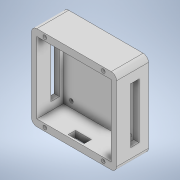
# Autodesk Inventor part: Case_Base
Saved by Autodesk Inventor 2022 (Build 260153000, 153)
## iProperties
Created: 2024-06-23
Part Number: Case_Base
Material: Типовые
Document SubType Name: Modeling
Designer: Timur
Density: 1 g/cm^3
Appearance: По умолчанию
Author: Timur
Autodesk Inventor part; units mm, degrees
ref_plane "YZ Plane" through (0, 0, 0) normal (1, 0, 0) x (0, 1, 0)
ref_plane "XZ Plane" through (0, 0, 0) normal (0, 1, 0) x (-1, 0, 0)
ref_plane "XY Plane" through (0, 0, 0) normal (0, 0, 1) x (1, 0, 0)
sketch "Эскиз1" plane through (0, 0, 0) normal (0, 0, 1) x (1, 0, 0)
  circle A0 centre (0, 2.5) radius 1.1
  circle A1 centre (55, 2.5) radius 1.1
  circle A2 centre (0, 57.5) radius 1.1
  circle A3 centre (55, 57.5) radius 1.1
  line L0 (15.5, 60) -> (0, 60)
  line L1 (-2.5, 57.5) -> (-2.5, 2.5)
  line L2 (55, 60) -> (39.5, 60)
  line L3 (57.5, 2.5) -> (57.5, 57.5)
  line L4 (-2.5, 2.5) -> (-2.5, 0)
  line L5 (0, 60) -> (-2.5, 60)
  line L6 (-2.5, 60) -> (-2.5, 57.5)
  line L7 (39.5, 60) -> (15.5, 60)
  line L8 (57.5, 2.5) -> (57.5, 0)
  line L9 (57.5, 0) -> (-2.5, 0)
  line L10 (57.5, 57.5) -> (57.5, 60)
  line L11 (57.5, 60) -> (55, 60)
  line L12 (-7.5, 63.5411) -> (62.5, 63.5411)
  line L13 (62.5, 63.5411) -> (62.5, -3.5411)
  line L14 (62.5, -3.5411) -> (-7.5, -3.5411)
  line L15 (-7.5, -3.5411) -> (-7.5, 63.5411)
  line L16 (-7.5, 63.5411) -> (62.5, -3.5411) construction
  line L17 (62.5, 63.5411) -> (-7.5, -3.5411) construction
  point P0 (0, 0)
  point P1 (27.5, 30)
  dimension "d0" = 70
  constraints: 36 end point, 5 perpendicular, 4 centre point, 3 vertical, 2 horizontal, 2 midpoint, 2 parallel
  measures "d0" distance of L13.end L14.end
extrude "Выдавливание1" add sketch "Эскиз1" along normal blind 5 contours A0 | A1 | A2 | A3 | L7 L2 L11 L10 L3 L8 L9 L4 L1 L6 L5 L0 | L12 L13 L14 L15
sketch "Эскиз2" plane through (0, 0, 0) normal (0, 0, -1) x (-1, 0, 0)
  line L0 (7.5, 63.5411) -> (7.5, -3.5411) projected
  line L1 (-62.5, -3.5411) -> (-62.5, 63.5411) projected
  line L2 (-62.5, 63.5411) -> (7.5, 63.5411) projected
  line L3 (7.5, -3.5411) -> (-62.5, -3.5411) projected
  line L4 (12.5, 70) -> (-67.5, 70)
  line L5 (-67.5, 70) -> (-67.5, -10)
  line L6 (-67.5, -10) -> (12.5, -10)
  line L7 (12.5, -10) -> (12.5, 70)
  line L8 (12.5, 70) -> (-67.5, -10) construction
  line L9 (-67.5, 70) -> (12.5, -10) construction
  point P0 (0, 0)
  point P1 (-27.5, 30)
  dimension "d3" = 80
  dimension "d4" = 80
  constraints: 12 end point, 2 midpoint, 2 parallel, 1 horizontal, 1 perpendicular
  measures "d3" distance of L6.end L5.end
  measures "d4" distance of L5.end L4.end
extrude "Выдавливание2" add sketch "Эскиз2" against normal blind 30
sketch "Эскиз3" plane through (0, 0, 5) normal (0, 0, 1) x (1, 0, 0)
  circle A0 centre (55, 2.5) radius 1.75
  circle A1 centre (55, 57.5) radius 1.75
  circle A2 centre (0, 57.5) radius 1.75
  circle A3 centre (0, 2.5) radius 1.75
  point P0 (0, 0)
  dimension "d7" = 3.5
  dimension "d8" = 3.5
  dimension "d9" = 3.5
  dimension "d10" = 3.5
  constraints: 4 centre point, 4 coincident
  measures "d7" diameter of A0
  measures "d8" diameter of A1
  measures "d9" diameter of A2
  measures "d10" diameter of A3
extrude "Выдавливание3" cut sketch "Эскиз3" against normal blind 4
fillet "Сопряжение1" radius 5 4 edges at (67.5, -10, 15) (67.5, 70, 15) (-12.5, -10, 15) (-12.5, 70, 15)
sketch "Эскиз5" plane through (0, 0, 30) normal (0, 0, 1) x (1, 0, 0)
  circle A0 centre (0, 57.5) radius 1.75 projected
  line L0 (0, 57.5) -> (0, 63.5411)
  line L1 (62.5, 63.5411) -> (-7.5, 63.5411) projected
  line L2 (-7.5, 70) -> (62.5, 70) projected
  line L3 (0, 70) -> (0, 63.5411)
  circle A1 centre (55, 57.5) radius 1.75 projected
  line L4 (55, 57.5) -> (55, 63.5411)
  line L5 (55, 63.5411) -> (55, 70)
  circle A2 centre (55, 66.7706) radius 1.75
  circle A3 centre (0, 66.7706) radius 1.75
  circle A4 centre (55, 2.5) radius 1.75 projected
  line L6 (55, 2.5) -> (55, -3.5411)
  line L7 (62.5, -3.5411) -> (-7.5, -3.5411) projected
  line L8 (55, -3.5411) -> (55, -10)
  line L9 (62.5, -10) -> (-7.5, -10) projected
  circle A5 centre (0, 2.5) radius 1.75 projected
  line L10 (0, 2.5) -> (0, -3.5411)
  line L11 (0, -3.5411) -> (0, -10)
  circle A6 centre (55, -6.7706) radius 1.75
  circle A7 centre (0, -6.7706) radius 1.75
  point P0 (0, 0)
  dimension "d14" = 3.5
  dimension "d15" = 3.5
  dimension "d16" = 3.5
  dimension "d17" = 3.5
  constraints: 16 end point, 8 point on line, 4 centre point, 4 midpoint, 4 vertical, 1 perpendicular
  measures "d14" diameter of A2
  measures "d15" diameter of A3
  measures "d16" diameter of A6
  measures "d17" diameter of A7
extrude "Выдавливание4" cut sketch "Эскиз5" against normal blind 4 contours A3 L3 | L3 A3 | A2 L5 | L5 A2 | A6 L8 | L8 A6 | A7 L11 | L11 A7
sketch "Эскиз6" plane through (0, 0, 30) normal (0, 0, 1) x (1, 0, 0)
  line L0 (62.5, 70) -> (-7.5, 70) projected
  line L1 (-12.5, 65) -> (-12.5, -5) projected
  arc A0 (-7.5, 70) -> (-12.5, 65) centre (-7.5, 65) ccw projected
  arc A1 (67.5, 65) -> (62.5, 70) centre (62.5, 65) ccw projected
  line L2 (67.5, -5) -> (67.5, 65) projected
  arc A2 (62.5, -10) -> (67.5, -5) centre (62.5, -5) ccw projected
  line L3 (-7.5, -10) -> (62.5, -10) projected
  arc A3 (-12.5, -5) -> (-7.5, -10) centre (-7.5, -5) ccw projected
  circle A4 centre (0, 66.7706) radius 1.75 projected
  circle A5 centre (55, 66.7706) radius 1.75 projected
  circle A6 centre (55, -6.7706) radius 1.75 projected
  circle A7 centre (0, -6.7706) radius 1.75 projected
  line L4 (62.5, -3.5411) -> (-7.5, -3.5411) projected
  line L5 (-7.5, -3.5411) -> (-7.5, 63.5411) projected
  line L6 (-7.5, 63.5411) -> (62.5, 63.5411) projected
  line L7 (62.5, 63.5411) -> (62.5, -3.5411) projected
  point P0 (0, 0)
sketch "Эскиз7" plane through (67.5, -5, 0) normal (1, 0, 0) x (0, 0, -1)
  line L0 (-30, -5) -> (0, -5)
  line L1 (-30, 0) -> (-30, 70)
  line L2 (0, 75) -> (-30, 75)
  line L3 (0, 70) -> (0, 0)
  line L4 (-30, 35) -> (0, 35)
  line L5 (-12.99, 13.983) -> (-12.99, 13.543)
  line L6 (-12.55, 13.543) -> (-12.55, 13.983)
  line L7 (-12.99, 13.763) -> (-12.55, 13.763)
  line L8 (-13.44, 12.493) -> (-12.1, 12.493)
  line L9 (-16.77, 9) -> (-8.77, 9)
  line L10 (-8.77, 9) -> (-8.77, 61)
  line L11 (-8.77, 61) -> (-16.77, 61)
  line L12 (-16.77, 61) -> (-16.77, 9)
  line L13 (-12.77, 13.763) -> (-12.77, 10.2135)
  point P0 (0, 5)
  dimension "d20" = 26
  dimension "d21" = 26
  dimension "d22" = 8
  dimension "d23" = 4
  constraints: 28 end point, 5 midpoint, 2 parallel, 1 horizontal, 1 perpendicular, 1 vertical
  measures "d20" distance between parallel lines of L4 L9
  measures "d21" distance between parallel lines of L4 L11
  measures "d22" distance between parallel lines of L10 L12
  measures "d23" distance between parallel lines of L13 L12
extrude "Выдавливание5" cut sketch "Эскиз7" against normal through all
sketch "Эскиз8" plane through (-7.5, -10, 0) normal (0, -1, 0) x (1, 0, 0)
  line L0 (32, 26.125) -> (38, 26.125)
  line L1 (34.72, 23.225) -> (32.7, 23.225)
  line L2 (30.9, 24.9) -> (30.9, 25.1)
  line L3 (39.1, 25.1) -> (39.1, 24.9)
  line L4 (30.9, 25.1) -> (30.9, 26.125)
  line L5 (30.9, 26.125) -> (39.1, 26.125)
  line L6 (39.1, 26.125) -> (39.1, 23.225)
  line L7 (39.1, 23.225) -> (30.9, 23.225)
  line L8 (30.9, 23.225) -> (30.9, 25.1)
  line L9 (42.5, 20.675) -> (27.5, 20.675)
  line L10 (27.5, 20.675) -> (27.5, 28.675)
  line L11 (27.5, 28.675) -> (42.5, 28.675)
  line L12 (42.5, 28.675) -> (42.5, 20.675)
  line L13 (42.5, 20.675) -> (27.5, 28.675) construction
  line L14 (27.5, 20.675) -> (42.5, 28.675) construction
  line L15 (42.5, 21.175) -> (27.5, 21.175)
  line L16 (27.5, 21.175) -> (27.5, 28.175)
  line L17 (27.5, 28.175) -> (42.5, 28.175)
  line L18 (42.5, 28.175) -> (42.5, 21.175)
  line L19 (42.5, 21.175) -> (27.5, 28.175) construction
  line L20 (27.5, 21.175) -> (42.5, 28.175) construction
  point P0 (7.5, 0)
  point P1 (35, 24.675)
  dimension "d26" = 15
  dimension "d27" = 8
  dimension "d28" = 15
  dimension "d29" = 7
  constraints: 42 end point, 5 perpendicular, 4 midpoint, 4 parallel, 2 horizontal, 2 point on line, 1 vertical
  measures "d26" distance of L10.end L11.end
  measures "d27" distance of L9.end L10.end
  measures "d28" distance of L16.end L17.end
  measures "d29" distance of L15.end L16.end
extrude "Выдавливание6" cut sketch "Эскиз8" against normal blind 10 contours L0 L5 L6 L3 L7 L1 L8 L2 L4 | L15 L10 L17 L12
